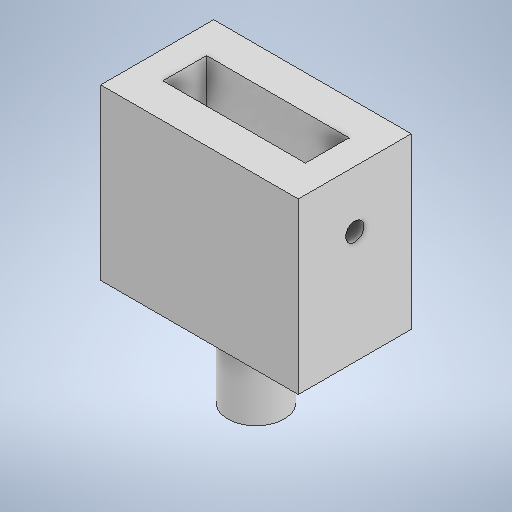
# Autodesk Inventor part: Idler_Klemme
Saved by Autodesk Inventor 2025 (Build 290162000, 162)
## iProperties
Created: 2026-07-09
Part Number: Idler_Klemme
Material: Generisch
Document SubType Name: Modeling
Designer: wavid
Mass: 9.30993 g
Surface Area: 42.974 cm^2
Volume: 9.30993 cm^3
Density: 1 g/cm^3
Appearance: Vorgabe
Author: wavid
Autodesk Inventor part; units mm, degrees
ref_plane "YZ Plane" through (0, 0, 0) normal (1, 0, 0) x (0, 1, 0)
ref_plane "XZ Plane" through (0, 0, 0) normal (0, 1, 0) x (-1, 0, 0)
sketch "Skizze1" plane through (0, 0, 0) normal (0, 0, 1) x (1, 0, 0)
  line L0 (-14, -8) -> (14, -8)
  line L1 (14, -8) -> (14, 8)
  line L2 (14, 8) -> (-14, 8)
  line L3 (-14, 8) -> (-14, -8)
  constraints: 8 end point, 2 parallel, 1 horizontal, 1 perpendicular
extrude "Extrusion1" add sketch "Skizze1" along normal blind 24
sketch "Skizze2" plane through (0, 0, 0) normal (0, 0, 1) x (1, 0, 0)
  circle A0 centre (0, 0) radius 4
  constraints: 1 centre point
extrude "Extrusion2" add sketch "Skizze2" against normal blind 12 separate body
ref_plane "Arbeitsebene1" through (0, 0, 24) normal (0, 0, 1) x (1, 0, 0)
sketch "Skizze3" plane through (0, 0, 24) normal (0, 0, 1) x (1, 0, 0)
  line L0 (-10.1, -3.1) -> (10.1, -3.1)
  line L1 (10.1, -3.1) -> (10.1, 3.1)
  line L2 (10.1, 3.1) -> (-10.1, 3.1)
  line L3 (-10.1, 3.1) -> (-10.1, -3.1)
  constraints: 8 end point, 2 parallel, 1 horizontal, 1 perpendicular
extrude "Extrusion3" cut sketch "Skizze3" against normal blind 16 bodies 1
sketch "Skizze4" plane through (0, 0, 0) normal (1, 0, 0) x (0, 1, 0)
  circle A0 centre (0, 16) radius 1.3
  constraints: 1 centre point
extrude "Extrusion4" cut sketch "Skizze4" along normal mid plane 30 bodies 1
